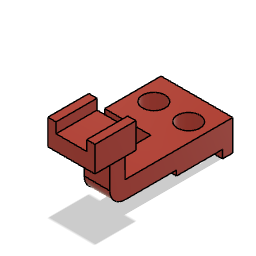
3d17 v1 (Autodesk Fusion 360 design; units mm, degrees)
Autodesk Fusion 360 part; units mm, degrees
sketch "Sketch1" plane through (0, 0, 0) normal (0, 1, 0) x (1, 0, 0)
  line L0 (0, 3.2328) -> (70, 3.2328)
  line L1 (70, 3.2328) -> (70, -51.7672)
  line L2 (70, -51.7672) -> (0, -51.7672)
  line L3 (0, -51.7672) -> (0, 3.2328)
  dimension "d1" = 70
  dimension "d2" = 55
  dimension "d3" = 55
  constraint horizontal L0
  constraint vertical L1
  constraint horizontal L2
  constraint vertical L3
  measures "d1" distance of L0.start L0.end
  measures "d2" distance of L0.start L2.end
  measures "d3" distance of L0.start L2.end
extrude "Extrude1" add sketch "Sketch1" along normal mid plane 30
sketch "Sketch2" plane through (70, 0, 0) normal (1, 0, 0) x (0, 0, -1)
  line L0 (3.2328, -15) -> (3.2328, 15)
  line L1 (3.2328, 15) -> (-51.7672, 15)
  line L2 (-51.7672, 15) -> (-51.7672, -15)
  line L3 (-51.7672, -15) -> (3.2328, -15)
  line L4 (-6.7672, -15) -> (-6.7672, -7)
  line L5 (-6.7672, -7) -> (-51.7672, -7)
  dimension "d6" = 10
  dimension "d7" = 45
  dimension "d8" = 8
  constraint coincident L3 L4.start
  constraint perpendicular L3 L4
  constraint coincident L2 L5.end
  constraint perpendicular L2 L5
  measures "d6" distance of L0.start L4.start
  measures "d7" distance of L4.end L5.end
  measures "d8" distance of L4.start L4.end
extrude "Extrude2" cut sketch "Sketch2" against normal blind 90 contours L2 L3 L4 L5
sketch "Sketch3" plane through (0, 15, 0) normal (0, 1, 0) x (-1, 0, 0)
  line L0 (0, 51.7672) -> (-70, 51.7672)
  line L1 (-70, 51.7672) -> (-70, -3.2328)
  line L2 (-70, -3.2328) -> (0, -3.2328)
  line L3 (0, -3.2328) -> (0, 51.7672)
  circle A0 centre (-18, 21.7672) radius 11
  circle A1 centre (-52, 21.7672) radius 11
  dimension "d11" = 22
  dimension "d12" = 22
  dimension "d13" = 30
  dimension "d14" = 18
  dimension "d15" = 34
  constraint horizontal A0.centre A1.centre
  measures "d11" diameter of A0
  measures "d12" diameter of A1
  measures "d13" vertical distance of L0.end A0.centre
  measures "d14" distance of L3 A0.centre
  measures "d15" distance of A0.centre A1.centre
extrude "Extrude3" cut sketch "Sketch3" against normal blind 50 contours A0 | A1
sketch "Sketch4" plane through (0, 15, 0) normal (0, 1, 0) x (-1, 0, 0)
  circle A0 centre (-52, 21.7672) radius 11
  circle A1 centre (-18, 21.7672) radius 11
  line L0 (0, 51.7672) -> (-70, 51.7672)
  line L1 (-70, 51.7672) -> (-70, -3.2328)
  line L2 (-70, -3.2328) -> (0, -3.2328)
  line L3 (0, -3.2328) -> (0, 51.7672)
  line L4 (-45, 51.7672) -> (-45, 101.7672)
  line L5 (-45, 101.7672) -> (-70, 101.7672)
  line L6 (-70, 101.7672) -> (-70, 51.7672)
  dimension "d18" = 50
  dimension "d19" = 50
  dimension "d20" = 25
  constraint coincident L0 L4.start
  constraint perpendicular L0 L4
  constraint perpendicular L4 L5
  constraint coincident L0.end L1.start
  constraint perpendicular L5 L6
  measures "d18" distance of L5.end L0.end
  measures "d19" distance of L4.start L4.end
  measures "d20" distance of L4.end L5.end
extrude "Extrude4" add sketch "Sketch4" against normal blind 17 contours L0 L4 L5 L6
sketch "Sketch5" plane through (70, 0, 0) normal (1, 0, 0) x (0, 0, -1)
  line L0 (-51.7672, -7) -> (-6.7672, -7)
  line L1 (-6.7672, -7) -> (-6.7672, -15)
  line L2 (-6.7672, -15) -> (3.2328, -15)
  line L3 (3.2328, -15) -> (3.2328, 15)
  line L4 (3.2328, 15) -> (-101.7672, 15)
  line L5 (-101.7672, 15) -> (-101.7672, -2)
  line L6 (-101.7672, -2) -> (-51.7672, -2)
  line L7 (-51.7672, -2) -> (-51.7672, -7)
  line L8 (-170, 80) -> (-115.9179, 80)
  line L9 (-170, 60) -> (-114.0006, 60)
  line L10 (-116.7673, 45) -> (-116.7673, 13)
  arc A0 (-116.7673, 13) -> (-101.7672, -2) centre (-101.7673, 13) ccw
  line L11 (-116.7673, 45) -> (-102.1531, 45)
  line L12 (-102.1531, 45) -> (-101.7672, 15)
  dimension "d25" = 32
  dimension "d26" = 15
  dimension "d27" = 30
  constraint horizontal L8
  constraint horizontal L9
  constraint vertical L10
  constraint coincident L5.end L6.start
  constraint perpendicular L10 L11
  constraint coincident L4.end L5.start
  constraint tangent L10 A0
  measures "d25" distance of L10.start L10.end
  measures "d26" radius of A0
  measures "d27" vertical distance of L11.end L4.end
extrude "Extrude5" add sketch "Sketch5" against normal blind 25 contours L5 L10 A0 L11 L12
sketch "Sketch6" plane through (0, 0, 116.7673) normal (0, 0, 1) x (1, 0, 0)
  line L0 (70, 13) -> (70, 45)
  line L1 (70, 45) -> (45, 45)
  line L2 (45, 45) -> (45, 13)
  line L3 (45, 13) -> (70, 13)
  line L4 (45, 45) -> (34.5, 45)
  line L5 (34.5, 45) -> (34.5, 70)
  line L6 (34.5, 70) -> (42.5, 70)
  line L7 (42.5, 70) -> (42.5, 60)
  line L8 (42.5, 60) -> (72.5, 60)
  line L9 (72.5, 60) -> (72.5, 70)
  line L10 (72.5, 70) -> (80.5, 70)
  line L11 (80.5, 70) -> (80.5, 45)
  line L12 (80.5, 45) -> (70, 45)
  dimension "d30" = 25
  dimension "d31" = 8
  dimension "d32" = 8
  dimension "d33" = 25
  dimension "d34" = 10.5
  dimension "d35" = 10.5
  dimension "d36" = 30
  dimension "d37" = 46
  constraint coincident L1.end L2.start
  constraint perpendicular L2 L4
  constraint perpendicular L4 L5
  constraint perpendicular L5 L6
  constraint perpendicular L6 L7
  constraint perpendicular L7 L8
  constraint perpendicular L6 L9
  constraint perpendicular L7 L10
  constraint perpendicular L10 L11
  constraint coincident L0.end L1.start
  constraint horizontal L11.end L0.end
  measures "d30" distance of L10.end L11.end
  measures "d31" distance of L9.end L10.end
  measures "d32" distance of L5.end L6.end
  measures "d33" distance of L4.end L5.end
  measures "d34" distance of L1.end L4.end
  measures "d35" horizontal distance of L11.end L0.end
  measures "d36" distance of L7.end L8.end
  measures "d37" horizontal distance of L4.end L11.end
extrude "Extrude6" add sketch "Sketch6" along normal blind 25 and the other way blind 15 contours L1 L4 L5 L6 L7 L8 L9 L10 L11 L12
